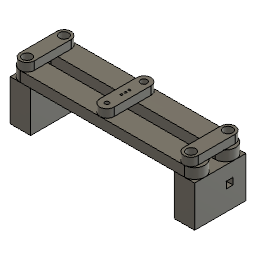
Ackerman System vinfinity (Autodesk Fusion 360 design; units mm, degrees)
Autodesk Fusion 360 part; units mm, degrees
note: some values were not read from the file. Chosen so that the rebuilt part matches the saved one: which face or edge a step refers to; which pieces of a blend or face edit are solid.
sketch "Sketch1" plane through (0, 0, 0) normal (0, 1, 0) x (1, 0, 0)
sketch "Sketch2" plane through (0, 0, 0) normal (0, 1, 0) x (1, 0, 0)
  line L0 (-35, -15) -> (-45, -15)
  line L1 (-45, -15) -> (-45, 10)
  line L2 (-45, 10) -> (-35, 10)
  line L3 (-35, 10) -> (-35, -15)
  line L4 (25, 10) -> (35, 10)
  line L5 (35, 10) -> (35, -15)
  line L6 (35, -15) -> (25, -15)
  line L7 (25, -15) -> (25, 10)
  line L8 (-45, 10) -> (35, 10)
  line L9 (35, 10) -> (35, 0)
  line L10 (35, 0) -> (-45, 0)
  line L11 (-45, 0) -> (-45, 10)
  line L12 (-45, -15) -> (35, -15)
  line L13 (35, -15) -> (35, -5)
  line L14 (35, -5) -> (-45, -5)
  line L15 (-45, -5) -> (-45, -15)
  line L16 (-42.7258, 10) -> (-37.7258, 10)
  line L17 (-37.7258, 10) -> (-37.7258, -15)
  line L18 (-37.7258, -15) -> (-42.7258, -15)
  line L19 (-42.7258, -15) -> (-42.7258, 10)
  line L20 (32.7117, 10) -> (27.7117, 10)
  line L21 (27.7117, 10) -> (27.7117, -15)
  line L22 (27.7117, -15) -> (32.7117, -15)
  line L23 (32.7117, -15) -> (32.7117, 10)
  line L24 (-7.1426, 10) -> (-1.1426, 10)
  line L25 (-1.1426, 10) -> (-1.1426, -15)
  line L26 (-1.1426, -15) -> (-7.1426, -15)
  line L27 (-7.1426, -15) -> (-7.1426, 10)
  line L28 (-37.7258, -15) -> (-44.7258, -15)
  line L29 (-44.7258, -15) -> (-44.7258, -40)
  line L30 (-44.7258, -40) -> (-37.7258, -40)
  line L31 (-37.7258, -40) -> (-37.7258, -15)
  dimension "d5" = 10
  dimension "d6" = 25
  dimension "d10" = 10
  dimension "d11" = 25
  dimension "d14" = 80
  dimension "d15" = 10
  dimension "d16" = 80
  dimension "d17" = 10
  dimension "d18" = 5
  dimension "d19" = 5
  dimension "d20" = 25
  dimension "d21" = 6
  dimension "d135" = 7
  dimension "d136" = 25
  constraint horizontal L0
  constraint vertical L1
  constraint horizontal L2
  constraint vertical L3
  constraint horizontal L4
  constraint vertical L5
  constraint horizontal L6
  constraint vertical L7
  constraint horizontal L8
  constraint vertical L9
  constraint horizontal L10
  constraint vertical L11
  constraint horizontal L12
  constraint vertical L13
  constraint horizontal L14
  constraint vertical L15
  constraint horizontal L16
  constraint vertical L17
  constraint horizontal L18
  constraint vertical L19
  constraint coincident L8 L16.start
  constraint horizontal L20
  constraint vertical L21
  constraint horizontal L22
  constraint vertical L23
  constraint coincident L8 L20.start
  constraint horizontal L24
  constraint vertical L25
  constraint horizontal L26
  constraint vertical L27
  constraint coincident L8 L24.start
  constraint horizontal L28
  constraint vertical L29
  constraint horizontal L30
  constraint vertical L31
  measures "d5" distance of L0.start L0.end
  measures "d6" distance of L0.start L2.end
  measures "d10" distance of L4.start L4.end
  measures "d11" distance of L4.start L6.end
  measures "d14" distance of L1.end L4.end
  measures "d15" distance of L1.end L10.end
  measures "d16" distance of L0.end L5.end
  measures "d17" distance of L0.end L14.end
  measures "d18" distance of L16.start L16.end
  measures "d19" distance of L20.start L20.end
  measures "d20" distance of L20.start L22.end
  measures "d21" distance of L24.start L24.end
  measures "d135" distance of L17.end L28.end
  measures "d136" distance of L17.end L30.end
extrude "Extrude2" add sketch "Sketch2" along normal blind 20 contours L0 L3 L12 L14 L17 | L0 L12 L14 L17 L18 L19 L28 | L3 L10 L14 L17 | L0 L1 L12 L14 L15 L19 L28 | L10 L14 L17 L19 | L2 L3 L8 L10 L17 | L1 L10 L14 L19 | L2 L8 L10 L16 L17 L19 | L1 L2 L8 L10 L11 L19 makes body 1
move_face "MoveFace1" by (0, -5, 0) 1 faces at (-38.3333, 20, 6.6667) on bodies 1
extrude "Extrude3" add sketch "Sketch2" along normal blind 20 separate body contours L6 L7 L12 L14 L21 | L7 L10 L14 L21 | L6 L12 L14 L21 L22 L23 | L4 L7 L8 L10 L21 | L10 L14 L21 L23 | L5 L6 L12 L13 L14 L23 | L4 L8 L10 L20 L21 L23 | L5 L10 L14 L23 | L4 L5 L8 L9 L10 L23 makes body 2
move_face "MoveFace3" by (0, 5, 0) 1 faces at (-38.3333, 15, 6.6667) on bodies 1
extrude "Extrude4" add sketch "Sketch2" along normal blind 5 separate body contours L0 L3 L12 L14 L17 | L3 L12 L14 L27 | L0 L12 L14 L17 L18 L19 L28 | L12 L14 L25 L26 L27 | L0 L1 L12 L14 L15 L19 L28 | L2 L3 L8 L10 L17 | L3 L8 L10 L27 | L7 L12 L14 L25 | L2 L8 L10 L16 L17 L19 | L8 L10 L24 L25 L27 | L6 L7 L12 L14 L21 | L1 L2 L8 L10 L11 L19 | L7 L8 L10 L25 | L6 L12 L14 L21 L22 L23 | L4 L7 L8 L10 L21 | L5 L6 L12 L13 L14 L23 | L4 L8 L10 L20 L21 L23 | L4 L5 L8 L9 L10 L23 makes body 3 at (-18.3333, 0, -3.3333) makes body 4 at (-18.3333, 0, 11.6667)
move_body "Move1" bodies 3 to x (1, 0, 0) y (0, 1, 0) z (0, 0, 1) at (0, 20, 0)
move_body "Move2" bodies 4 to x (1, 0, 0) y (0, 1, 0) z (0, 0, 1) at (0, 20, 0)
fillet "Fillet3" radius 5 1 edges at (35, 22.5, -10) on bodies 3
fillet "Fillet4" radius 5 1 edges at (35, 22.5, 0) on bodies 3
fillet "Fillet5" radius 5 1 edges at (35, 22.5, 15) on bodies 4
fillet "Fillet6" radius 5 1 edges at (35, 22.5, 5) on bodies 4
hole "Hole7" at (35, 10, 2.5) direction (-1, 0, 0) diameter 3 depth 10 tip angle 118 bodies 2
hole "Hole8" at (-45, 10, 2.5) direction (1, 0, 0) diameter 3 depth 16 tip angle 118 bodies 1
sketch "Sketch4" plane through (0, 0, 0) normal (0, 1, 0) x (1, 0, 0)
  point P0 (-40.221, 5.5863)
  point P1 (-40.221, -10.8439)
  point P2 (-4.9948, -10.8439)
  point P3 (-5.0901, 5.5863)
  point P4 (30.2677, 5.5863)
  point P5 (30.2677, -11.261)
sketch "Sketch5" plane through (0, 0, 0) normal (0, 1, 0) x (1, 0, 0)
sketch "Sketch6" plane through (0, 0, 0) normal (0, 1, 0) x (1, 0, 0)
move_body "Move18" bodies 1 to x (1, 0, 0) y (0, 1, 0) z (0, 0, 1) at (-10, 0, 0)
move_face "MoveFace10" by (-10, 0, 0) 1 faces at (-45, 21.6667, -3.3333) on bodies 3
move_face "MoveFace11" by (-10, 0, 0) 1 faces at (-45, 21.6667, 11.6667) on bodies 4
fillet "Fillet14" radius 5 1 edges at (-55, 22.5, 15) on bodies 4
fillet "Fillet15" radius 5 1 edges at (-55, 22.5, 5) on bodies 4
fillet "Fillet16" radius 5 1 edges at (-55, 22.5, 0) on bodies 3
fillet "Fillet17" radius 5 1 edges at (-55, 22.5, -10) on bodies 3
extrude "Extrude6" add sketch "Sketch2" along normal blind 4 separate body contours L0 L12 L18 L28 L29 L30 L31 makes body 5
fillet "Fillet18" radius 3.5 1 edges at (-44.7258, 2, 40) on bodies 5
fillet "Fillet19" radius 3.5 1 edges at (-37.7258, 2, 40) on bodies 5
fillet "Fillet20" radius 3.5 1 edges at (-44.7258, 2, 15) on bodies 5
fillet "Fillet21" radius 3.5 1 edges at (-37.7258, 2, 15) on bodies 5
move_body "Move32" bodies 5 to x (1, 0, 0) y (0, 1, 0) z (0, 0, 1) at (15, 25, -10)
move_body "Move34" bodies 5 to x (1, 0, 0) y (0, 1, 0) z (0, 0, 1) at (-22.5, 0, 0)
move_body "Move35" bodies 5 to x (1, 0, 0) y (0, 1, 0) z (0, 0, 1) at (0, 0, -15)
move_body "Move36" bodies 5 to x (1, 0, 0) y (0, 1, 0) z (0, 0, 1) at (-1.5, 0, 0)
hole "Hole26" at (-50.2258, 29, 11.5) direction (0, -1, 0) diameter 4.5 depth 33 tip angle 118 bodies 1 4 5
copy_body "CopyPasteBodies1" bodies 5 makes body 6
move_body "Move37" bodies 6 to x (1, 0, 0) y (0, 1, 0) z (0, 0, 1) at (0, 0, 0)
move_body "Move38" bodies 6 to x (1, 0, 0) y (0, 1, 0) z (0, 0, 1) at (80, 0, 0)
hole "Hole27" at (-50.2258, 29, -6.5) direction (0, -1, 0) diameter 4.5 depth 66 tip angle 118 bodies 3 5
hole "Hole28" at (-50.3096, 20, -6.5729) direction (0, -1, 0) diameter 4.5 depth 24 tip angle 118 bodies 1
delete_face "DeleteFace1" 1 faces at (29.9983, 26.3333, 13.7388) on bodies 6
hole "Hole29" at (29.7742, 29, 11.5) direction (0, -1, 0) diameter 4.5 depth 34 tip angle 118 bodies 2 4 6
hole "Hole30" at (29.7742, 29, -6.5) direction (0, -1, 0) diameter 4.5 depth 44 tip angle 118 bodies 2 3 6
copy_body "CopyPasteBodies2" bodies 6 makes body 7
move_body "Move39" bodies 7 to x (1, 0, 0) y (0, 1, 0) z (0, 0, 1) at (0, 0, 0)
move_body "Move40" bodies 7 to x (1, 0, 0) y (0, 1, 0) z (0, 0, 1) at (-35, 0, 0)
move_body "Move41" bodies 7 to x (1, 0, 0) y (0, 1, 0) z (0, 0, 1) at (-6, 0, 0)
delete_face "DeleteFace2" 1 faces at (-11.0017, 26.3333, 13.7388) on bodies 7
delete_face "DeleteFace3" 1 faces at (-11.1136, 27.6667, -4.2528) on bodies 7
hole "Hole31" at (-11.2258, 29, 11.5) direction (0, -1, 0) diameter 2 depth 44 tip angle 118 bodies 4 7
hole "Hole32" at (-11.2258, 29, -6.5) direction (0, -1, 0) diameter 3.2 depth 44 tip angle 118 bodies 3 7
hole "Hole33" at (-11.1924, 29, 9.8457) direction (0, -1, 0) diameter 0.5 depth 4 tip angle 118 bodies 4 7
hole "Hole34" at (-11.2252, 29, 9.0875) direction (0, -1, 0) diameter 0.5 depth 4 tip angle 118 bodies 4 7
hole "Hole35" at (-11.2475, 29, 8.2974) direction (0, -1, 0) diameter 0.5 depth 4 tip angle 118 bodies 4 7
copy_body "CopyPasteBodies3" bodies 7 makes body 8
move_body "Move42" bodies 8 to x (1, 0, 0) y (0, 1, 0) z (0, 0, 1) at (0, 0, 0)
move_face "MoveFace13" to x (1, 0, 0) y (0, 1, 0) z (0, 0, 1) at (-0.025, 0, 0) 1 faces at (-11.2497, 24.9666, 9.6599) on bodies 4
hole "Hole36" at (-11.2599, 29, 7.4996) direction (0, -1, 0) diameter 0.5 depth 4 tip angle 118 bodies 4 7 8
move_face "MoveFace14" to x (1, 0, 0) y (0, 1, 0) z (0, 0, 1) at (1, 0, 0) 1 faces at (-11.2747, 24.9666, 9.6599) on bodies 4
delete_face "DeleteFace4" 1 faces at (-10.2747, 24.9666, 9.6599) on bodies 4
hole "Hole37" at (-11.2533, 29, 6.7529) direction (0, -1, 0) diameter 0.5 depth 4 tip angle 118 bodies 4 7
hole "Hole38" at (-11.2274, 29, 7.4996) direction (0, -1, 0) diameter 0.5 depth 4 tip angle 118 bodies 7
hole "Hole39" at (-11.2351, 29, 5.9859) direction (0, -1, 0) diameter 0.5 depth 4 tip angle 118 bodies 7
hole "Hole40" at (-11.2302, 29, 9.8457) direction (0, -1, 0) diameter 0.5 depth 4 tip angle 118 bodies 7
delete_face "DeleteFace6" 1 faces at (-11.1379, 27.6667, 5.7555) on bodies 7
delete_face "DeleteFace7" 1 faces at (-11.1561, 27.6667, 6.5226) on bodies 7
delete_face "DeleteFace8" 1 faces at (-11.0611, 27.6667, 7.313) on bodies 7
delete_face "DeleteFace9" 1 faces at (-11.1628, 27.6667, 7.2693) on bodies 7
delete_face "DeleteFace10" 1 faces at (-11.3778, 27.6667, 8.0841) on bodies 7
delete_face "DeleteFace11" 1 faces at (-11.3097, 26.3333, 10.0827) on bodies 7
delete_face "DeleteFace12" 1 faces at (-11.312, 27.6667, 9.6261) on bodies 7
delete_face "DeleteFace13" 1 faces at (-11.3556, 27.6667, 8.8741) on bodies 7
hole "Hole41" at (-11.2258, 29, 2.5) direction (0, -1, 0) diameter 1 depth 4 tip angle 118 bodies 7
hole "Hole42" at (-11.1687, 29, 4.5042) direction (0, -1, 0) diameter 1 depth 4 tip angle 118 bodies 4 7
hole "Hole43" at (-11.1734, 29, 0.6104) direction (0, -1, 0) diameter 1 depth 4 tip angle 118 bodies 7
delete_face "DeleteFace14" 1 faces at (31.6667, 10.0748, 1.0019) on bodies 2
delete_face "DeleteFace15" 1 faces at (-51.6667, 10.0748, 3.9981) on bodies 1
hole "Hole44" at (35, 13.1574, 1.8208) direction (-1, 0, 0) diameter 1 depth 4 tip angle 118 bodies 2
delete_face "DeleteFace16" 1 faces at (33.6667, 13.1823, 1.3214) on bodies 2
sketch "Sketch8" plane through (35, 0, 0) normal (1, 0, 0) x (0, 0, -1)
  line L0 (10, 20) -> (-15, 20)
  line L1 (-15, 20) -> (-15, 0)
  line L2 (-15, 0) -> (10, 0)
  line L3 (10, 0) -> (10, 20)
  line L4 (0.5, 13) -> (3.7, 13)
  line L5 (3.7, 13) -> (3.7, 9.8)
  line L6 (3.7, 9.8) -> (0.5, 9.8)
  line L7 (0.5, 9.8) -> (0.5, 13)
  line L8 (3.7, 10.8711) -> (10, 10.8711)
  line L9 (2.1, 9.8) -> (2.1, 0)
  dimension "d209" = 3.2
  dimension "d210" = 3.2
  constraint horizontal L4
  constraint vertical L5
  constraint horizontal L6
  constraint vertical L7
  constraint coincident L5 L8.start
  constraint coincident L3 L8.end
  constraint perpendicular L3 L8
  constraint midpoint L6 L9.start
  constraint coincident L2 L9.end
  constraint perpendicular L2 L9
  measures "d209" distance of L4.start L4.end
  measures "d210" distance of L4.start L6.end
sketch "Sketch9" plane through (35, 0, 0) normal (1, 0, 0) x (0, 0, -1)
sketch "Sketch10" plane through (-55, 0, 0) normal (-1, 0, 0) x (0, 0, 1)
  line L0 (-10, 0) -> (15, 0)
  line L1 (15, 0) -> (15, 20)
  line L2 (15, 20) -> (-10, 20)
  line L3 (-10, 20) -> (-10, 0)
  line L4 (-3.6847, 13.0058) -> (-0.4847, 13.0058)
  line L5 (-0.4847, 13.0058) -> (-0.4847, 9.8058)
  line L6 (-0.4847, 9.8058) -> (-3.6847, 9.8058)
  line L7 (-3.6847, 9.8058) -> (-3.6847, 13.0058)
  line L8 (15, 13) -> (12.7, 13)
  line L9 (-10, 13.0058) -> (-3.7, 13.0058)
  line L10 (-1.31, 9.8058) -> (-1.31, 0)
  dimension "d211" = 3.2
  dimension "d212" = 3.2
  dimension "d222" = 6.3
  constraint horizontal L4
  constraint vertical L5
  constraint horizontal L6
  constraint vertical L7
  constraint coincident L1 L8.start
  constraint perpendicular L1 L8
  constraint coincident L3 L9.start
  constraint perpendicular L7 L9
  constraint coincident L6 L10.start
  constraint coincident L0 L10.end
  constraint perpendicular L0 L10
  measures "d211" distance of L4.start L4.end
  measures "d212" distance of L4.start L6.end
  measures "d222" distance of L9.start L9.end
extrude "Extrude9" cut sketch "Sketch8" against normal blind 10 contours L4 L5 L6 L7 bodies 2
extrude "Extrude10" cut sketch "Sketch10" against normal blind 10 contours L4 L5 L6 L7 bodies 1
move_body "Move49" [rolled back]
hidden bodies 8
